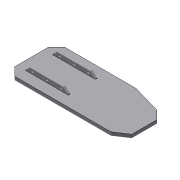
# Autodesk Inventor part: Left foot
Saved by Autodesk Inventor 2011 (Build 150239000, 239)
## iProperties
Created: 2010-11-21
Part Number: Left foot
Document SubType Name: Modeling
Designer: Milton
Density: 2.71 g/cm^3
Mass: 88.8482 g
Surface Area: 183.661 cm^2
Volume: 32.7853 cm^3
Material: Aluminum-6061
Author: Milton
Autodesk Inventor part; units mm, degrees
ref_plane "YZ Plane" through (0, 0, 0) normal (1, 0, 0) x (0, 1, 0)
ref_plane "XZ Plane" through (0, 0, 0) normal (0, 1, 0) x (-1, 0, 0)
ref_plane "XY Plane" through (0, 0, 0) normal (0, 0, 1) x (1, 0, 0)
sketch "Sketch1" plane through (0, 0, 0) normal (0, 0, 1) x (1, 0, 0)
  line L0 (71.1315, 22.4272) -> (71.1315, 24.9272)
  line L1 (25.7315, 22.4272) -> (25.7315, 24.9272)
  line L2 (65.5315, 22.4272) -> (65.5315, 24.9272)
  line L3 (71.1315, 57.4272) -> (71.1315, 54.9272)
  line L4 (25.7315, 57.4272) -> (25.7315, 54.9272)
  line L5 (65.5315, 57.4272) -> (65.5315, 54.9272)
  line L6 (10.1315, 19.9272) -> (10.1315, 59.9272)
  line L7 (20.1315, 69.9272) -> (105.1315, 69.9272)
  line L8 (150.1315, 49.9272) -> (150.1315, 19.9272)
  line L9 (135.1315, 9.9272) -> (20.1315, 9.9272)
  line L10 (10.1315, 19.9272) -> (20.1315, 9.9272)
  line L11 (105.1315, 69.9272) -> (140.1315, 59.9272)
  line L12 (10.1315, 59.9272) -> (20.1315, 69.9272)
  line L13 (150.1315, 49.9272) -> (140.1315, 59.9272)
  line L14 (135.1315, 9.9272) -> (150.1315, 19.9272)
  line L15 (20.1315, 22.4272) -> (20.1315, 24.9272)
  line L16 (20.1315, 24.9272) -> (71.1315, 24.9272)
  line L17 (71.1315, 22.4272) -> (20.1315, 22.4272)
  line L18 (20.1315, 57.4272) -> (20.1315, 54.9272)
  line L19 (20.1315, 54.9272) -> (71.1315, 54.9272)
  line L20 (71.1315, 57.4272) -> (20.1315, 57.4272)
  constraints: 42 end point, 8 point on line
extrude "Extrusion1" add sketch "Sketch1" against normal blind 4 contours L17 L2 L16 L0 | L17 L1 L16 L2 | L17 L15 L16 L1 | L3 L19 L5 L20 | L5 L19 L4 L20 | L4 L19 L18 L20 | L6 L12 L7 L11 L13 L8 L14 L9 L10
extrude "Extrusion2" add sketch "Sketch1" along normal blind 5.6 contours L17 L2 L16 L0 | L17 L1 L16 L2 | L17 L15 L16 L1 | L3 L19 L5 L20 | L5 L19 L4 L20 | L4 L19 L18 L20
sketch "Sketch2" plane through (20.1315, 22.4272, 5.6) normal (0, -1, 0) x (1, 0, 0)
  line L0 (0, -5.6) -> (0, 0) projected
  circle A0 centre (8.5, -2.8) radius 1.35
  circle A1 centre (25.5, -2.8) radius 1.35
  circle A2 centre (42.5, -2.8) radius 1.35
  point P0 (-20.1315, -5.6)
  dimension "d5" = 2.7
  dimension "d6" = 2.7
  dimension "d7" = 2.7
  dimension "d8" = 17
  dimension "d9" = 17
  dimension "d10" = 8.5
  constraints: 3 centre point
  measures "d5" diameter of A0
  measures "d6" diameter of A1
  measures "d7" diameter of A2
  measures "d8" distance of A2.centre A1.centre
  measures "d9" distance of A0.centre A1.centre
  measures "d10" distance from line of L0 A0.centre
extrude "Extrusion3" cut sketch "Sketch2" against normal through all
chamfer "Chamfer1" distance 5.6 angle 45 4 edges at (20.1315, 23.6772, 5.6) (20.1315, 56.1772, 5.6) (71.1315, 23.6772, 5.6) (71.1315, 56.1772, 5.6)
body "Solid1"
